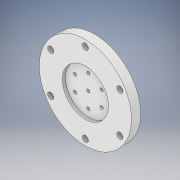
# Autodesk Inventor part: SJ002
Saved by Autodesk Inventor 2017 SP1 (Build 210196100, 196)
## iProperties
Created: 2017-06-01
Part Number: SJ002
Material: ABS Plastic
Document SubType Name: Modeling
Designer: Zach
Density: 1.06 g/cm^3
Appearance: CR White
Author: Zach
Autodesk Inventor part; units mm, degrees
ref_plane "YZ Plane" through (0, 0, 0) normal (1, 0, 0) x (0, 1, 0)
ref_plane "XZ Plane" through (0, 0, 0) normal (0, 1, 0) x (-1, 0, 0)
ref_plane "XY Plane" through (0, 0, 0) normal (0, 0, 1) x (1, 0, 0)
sketch "Sketch2" plane through (0, 0, 0) normal (0, 0, 1) x (1, 0, 0)
  circle A0 centre (0, 0) radius 75
  circle A1 centre (0, 0) radius 2.5
  dimension "d0" = 150
  dimension "d1" = 5
  constraints: 2 centre point, 2 coincident
  measures "d0" diameter of A0
  measures "d1" diameter of A1
extrude "Extrusion1" add sketch "Sketch2" along normal blind 15
sketch "Sketch4" plane through (0, 0, 0) normal (0, 0, -1) x (-1, 0, 0)
  circle A0 centre (0, 25) radius 2.575
  circle A1 centre (-21.6506, 12.5) radius 2.575
  circle A2 centre (-21.6506, -12.5) radius 2.575
  circle A3 centre (0, -25) radius 2.575
  circle A4 centre (21.6506, -12.5) radius 2.575
  circle A5 centre (21.6506, 12.5) radius 2.575
  point P0 (0, 0)
  dimension "d8" = 5.15
  dimension "d9" = 25
  dimension "d12" = 360
  constraints: 6 centre point, 1 vertical alignment, 13 other
  measures "d8" diameter of A0
  measures "d9" distance of point (0, 0) A0.centre
extrude "Extrusion3" cut sketch "Sketch4" against normal through all
sketch "Sketch5" plane through (0, 0, 15) normal (0, 0, 1) x (1, 0, 0)
  circle A0 centre (0, 0) radius 37.5
  dimension "d16" = 75
  constraints: 1 centre point, 1 coincident
  measures "d16" diameter of A0
extrude "Extrusion4" cut sketch "Sketch5" against normal blind 5
sketch "Sketch6" plane through (0, 0, 15) normal (0, 0, 1) x (1, 0, 0)
  circle A0 centre (0, 65) radius 2.5
  circle A1 centre (-56.2917, 32.5) radius 2.5
  circle A2 centre (-56.2917, -32.5) radius 2.5
  circle A3 centre (0, -65) radius 2.5
  circle A4 centre (56.2917, -32.5) radius 2.5
  circle A5 centre (56.2917, 32.5) radius 2.5
  point P0 (0, 0)
  dimension "d19" = 5
  dimension "d20" = 65
  dimension "d23" = 360
  constraints: 6 centre point, 13 other
  measures "d19" diameter of A0
  measures "d20" distance of point (0, 0) A0.centre
extrude "Extrusion5" cut sketch "Sketch6" against normal through all
sketch "Sketch8" plane through (0, 0, 15) normal (0, 0, 1) x (1, 0, 0)
  circle A0 centre (56.2917, -32.5) radius 2.5 projected
  circle A1 centre (-56.2917, -32.5) radius 2.5 projected
  circle A2 centre (0, 65) radius 2.5 projected
  circle A3 centre (-56.2917, 32.5) radius 2.5 projected
  circle A4 centre (0, -65) radius 2.5 projected
  circle A5 centre (56.2917, 32.5) radius 2.5 projected
  circle A6 centre (0, 0) radius 37.5 projected
  circle A7 centre (0, 0) radius 75 projected
  circle A8 centre (0, 65) radius 2.5 projected
  circle A9 centre (0, 65) radius 5
  circle A10 centre (-56.2917, 32.5) radius 5
  circle A11 centre (-56.2917, -32.5) radius 5
  circle A12 centre (0, -65) radius 5
  circle A13 centre (56.2917, -32.5) radius 5
  circle A14 centre (56.2917, 32.5) radius 5
  dimension "d28" = 10
  dimension "d31" = 360
  constraints: 6 centre point, 1 coincident, 19 other
  measures "d28" diameter of A9
extrude "Extrusion6" cut sketch "Sketch8" against normal blind 5 contours A9 | A10 | A11 | A12 | A13 | A14
body "Solid1"
